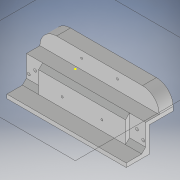
# Autodesk Inventor part: 000.001.010 - Realsense крепление
Saved by Autodesk Inventor 2022 (Build 260153000, 153)
## iProperties
Created: 2022-12-25
Part Number: 000.001.010 - Realsense крепление
Material: Типовые
Document SubType Name: Modeling
Designer: Ivan Petrov
Density: 1 g/cm^3
Appearance: По умолчанию
Author: Ivan Petrov
Autodesk Inventor part; units mm, degrees
ref_plane "YZ Plane" through (0, 0, 0) normal (1, 0, 0) x (0, 1, 0)
ref_plane "XZ Plane" through (0, 0, 0) normal (0, 1, 0) x (-1, 0, 0)
ref_plane "XY Plane" through (0, 0, 0) normal (0, 0, 1) x (1, 0, 0)
sketch "Эскиз1" plane through (0, 0, 0) normal (0, 0, 1) x (1, 0, 0)
  point P0 (0, 0)
sketch "Эскиз2" plane through (0, 0, 0) normal (1, 0, 0) x (0, 1, 0)
  line L0 (54.4194, 8.3986) -> (39.8994, 8.3986)
  line L1 (59.4094, -4.1014) -> (59.4094, 3.8986)
  line L2 (64.4094, 15.8986) -> (64.4094, -11.1014)
  line L3 (61.9094, 18.3986) -> (34.9094, 18.3986)
  line L4 (32.4094, 20.8986) -> (32.4094, 47.8986)
  line L5 (23.4094, 30.3986) -> (6.4094, 30.3986)
  line L6 (27.4094, 14.7056) -> (27.4094, 16.0719)
  line L7 (59.4094, -11.1014) -> (64.4094, -11.1014)
  line L8 (64.4094, -11.1014) -> (64.4094, 18.3986)
  line L9 (64.4094, 18.3986) -> (59.4094, 18.3986)
  line L10 (59.4094, 18.3986) -> (59.4094, -11.1014)
  line L11 (32.4094, 8.3986) -> (59.4094, 8.3986)
  line L12 (59.4094, 8.3986) -> (59.4094, 18.3986)
  line L13 (59.4094, 18.3986) -> (32.4094, 18.3986)
  line L14 (32.4094, 18.3986) -> (32.4094, 8.3986)
  line L15 (27.4094, 8.3986) -> (32.4094, 8.3986)
  line L16 (32.4094, 8.3986) -> (32.4094, 47.8986)
  line L17 (32.4094, 47.8986) -> (27.4094, 47.8986)
  line L18 (27.4094, 47.8986) -> (27.4094, 8.3986)
  line L19 (6.4094, 30.3986) -> (27.4094, 30.3986)
  line L20 (27.4094, 30.3986) -> (27.4094, 47.8986)
  line L21 (27.4094, 47.8986) -> (6.4094, 47.8986)
  line L22 (6.4094, 47.8986) -> (6.4094, 30.3986)
  point P0 (0, 0)
  point P1 (59.4094, 8.3986)
  point P2 (61.9094, 18.3986)
  point P3 (34.9094, 18.3986)
  point P4 (32.4094, 8.3986)
  point P5 (27.4094, 8.3986)
extrude "Выдавливание1" add sketch "Эскиз2" along normal mid plane 150
sketch "Эскиз3" plane through (75, 59.4094, 8.3986) normal (0, 0, -1) x (-1, 0, 0)
  circle A0 centre (147, -11) radius 1.85 projected
  circle A1 centre (3, -11) radius 1.85 projected
  circle A2 centre (11, -19) radius 1.85 projected
  circle A3 centre (139, -19) radius 1.85 projected
  point P0 (75, -59.4094)
extrude "Выдавливание2" cut sketch "Эскиз3" against normal through all
sketch "Эскиз4" plane through (75, 59.4094, 8.3986) normal (0, 0, -1) x (-1, 0, 0)
  line L0 (150, 0) -> (150, -32) projected
  line L1 (150, 0) -> (0, 0) projected
  line L2 (150, -32) -> (129.5965, -32)
  line L3 (129.5965, -32) -> (129.5965, 0)
  line L4 (129.5965, 0) -> (150, 0)
  line L5 (150, 0) -> (150, -32)
  line L6 (150, -32) -> (0, -32) projected
  point P0 (75, -59.4094)
  point P1 (139.7982, -32)
  constraints: 8 end point, 3 point on line, 2 parallel, 1 horizontal, 1 midpoint, 1 perpendicular
extrude "Выдавливание3" cut sketch "Эскиз4" against normal blind 5
mirror "Зеркальное отражение1" about plane through (0, 0, 0) normal (1, 0, 0) of "Выдавливание3"
sketch "Эскиз5" plane through (-75, 6.4094, 47.8986) normal (0, 0, 1) x (1, 0, 0)
  circle A0 centre (97.5, 8.5) radius 1.25 projected
  circle A1 centre (52.5, 8.5) radius 1.25 projected
  circle A2 centre (100, 40.75) radius 1.2645 projected
  circle A3 centre (50, 40.75) radius 1.2645 projected
  point P0 (75, -6.4094)
extrude "Выдавливание4" cut sketch "Эскиз5" against normal through all
sketch "Эскиз6" plane through (-75, 6.4094, 47.8986) normal (0, 0, 1) x (1, 0, 0)
  circle A0 centre (97.5, 8.5) radius 1.25 projected
  circle A1 centre (97.5, 8.5) radius 5
  circle A2 centre (52.5, 8.5) radius 1.25 projected
  circle A3 centre (52.5, 8.5) radius 5
  point P0 (75, -6.4094)
  dimension "d8" = 10
  dimension "d9" = 10
  constraints: 2 centre point, 2 coincident
  measures "d8" diameter of A1
  measures "d9" diameter of A3
extrude "Выдавливание5" cut sketch "Эскиз6" against normal blind 14.5 contours A0 | A1 | A2 | A3
sketch "Эскиз7" plane through (-75, 32.4094, 18.3986) normal (0, 0, 1) x (1, 0, 0)
  circle A0 centre (100, 14.75) radius 1.2645 projected
  circle A1 centre (100, 14.75) radius 5
  circle A2 centre (50, 14.75) radius 1.2645 projected
  circle A3 centre (50, 14.75) radius 5
  point P0 (75, -32.4094)
  dimension "d12" = 10
  dimension "d13" = 10
  constraints: 2 centre point, 2 coincident
  measures "d12" diameter of A1
  measures "d13" diameter of A3
extrude "Выдавливание6" cut sketch "Эскиз7" against normal blind 7 contours A0 | A1 | A2 | A3
fillet "Сопряжение1" radius 21 2 edges at (75, 6.4094, 39.1486) (-75, 6.4094, 39.1486)
chamfer "Фаска1" distance 5 angle 45 2 edges at (64.7982, 59.4094, 13.3986) (-64.7982, 59.4094, 13.3986)
chamfer "Фаска2" distance 5 angle 45 1 edges at (0, 27.4094, 8.3986)
